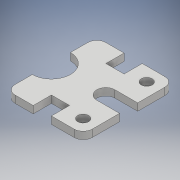
# Autodesk Inventor part: P2-6
Saved by Autodesk Inventor 2017 (Build 210142000, 142)
## iProperties
Created: 2017-02-09
Part Number: P2-6
Material: Generic
Document SubType Name: Modeling
Designer: Schaffel
Density: 1 g/cm^3
Appearance: Default
Author: Schaffel
Autodesk Inventor part; units mm, degrees
ref_plane "YZ Plane" through (0, 0, 0) normal (1, 0, 0) x (0, 1, 0)
ref_plane "XZ Plane" through (0, 0, 0) normal (0, 1, 0) x (-1, 0, 0)
ref_plane "XY Plane" through (0, 0, 0) normal (0, 0, 1) x (1, 0, 0)
sketch "Sketch1" plane through (0, 0, 0) normal (0, 0, 1) x (1, 0, 0)
  arc A0 (10, 100) -> (0, 90) centre (10, 90) ccw
  arc A1 (85, 90) -> (75, 100) centre (75, 90) ccw
  arc A2 (75, 0) -> (85, 10) centre (75, 10) ccw
  arc A3 (0, 10) -> (10, 0) centre (10, 10) ccw
  circle A4 centre (70, 15) radius 6
  circle A5 centre (70, 85) radius 6
  arc A6 (60, 60) -> (60, 40) centre (60, 50) ccw
  line L0 (60, 60) -> (85, 60)
  line L1 (60, 40) -> (85, 40)
  line L2 (30, 100) -> (30, 80)
  line L3 (30, 80) -> (50, 80)
  line L4 (50, 80) -> (50, 100)
  line L5 (30, 0) -> (30, 20)
  line L6 (30, 20) -> (50, 20)
  line L7 (50, 20) -> (50, 0)
  arc A7 (0, 29) -> (0, 71) centre (0, 50) ccw
  line L8 (0, 90) -> (0, 71)
  line L9 (0, 29) -> (0, 10)
  line L10 (75, 100) -> (50, 100)
  line L11 (30, 100) -> (10, 100)
  line L12 (85, 10) -> (85, 40)
  line L13 (85, 60) -> (85, 90)
  line L14 (10, 0) -> (30, 0)
  line L15 (50, 0) -> (75, 0)
  point P0 (0, 0)
  point P1 (85, 100)
  point P2 (85, 0)
  point P3 (0, 100)
  dimension "d0" = 85
  dimension "d1" = 100
  dimension "d2" = 10
  dimension "d3" = 10
  dimension "d4" = 10
  dimension "d5" = 10
  constraints: 32 end point, 16 tangent, 12 point on circle, 10 perpendicular, 8 centre point, 8 parallel, 4 point on line, 3 horizontal, 1 vertical
  measures "d0" distance of point (0, 100) point (85, 100)
  measures "d1" distance of point (85, 100) point (85, 0)
  measures "d2" radius of A0
  measures "d3" radius of A1
  measures "d4" radius of A2
  measures "d5" radius of A3
extrude "Extrusion1" add sketch "Sketch1" along normal blind 8
body "Solid1"
